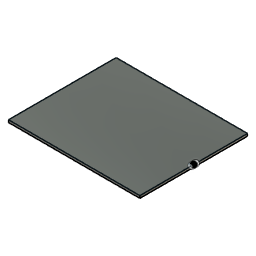
hydraulique (Autodesk Fusion 360 design; units mm, degrees)
Autodesk Fusion 360 part; units mm, degrees
box "BoxPrimitive1" add length 136 width 166 height 3 placed x (0, -1, 0) y (1, 0, 0) z (0, 0, 1) at (-30, 40, 0)
move_body "Move1" bodies 1 to x (1, 0, 0) y (0, 1, 0) z (0, 0, 1) at (-59.3373, 23.0424, 23.0424)
move_body "Move2" bodies 1 to x (1, 0, 0) y (0, 1, 0) z (0, 0, 1) at (6.3373, 4.9576, -26.0424)
move_body "Move3" bodies 1 to x (1, 0, 0) y (0, 1, 0) z (0, 0, 1) at (0, 0, 3)
sketch "Sketch6" plane through (0, 0, 3) normal (0, 0, 1) x (-1, 0, 0)
  line L0 (83, 68) -> (-83, 68)
  line L1 (-83, 68) -> (-83, -68)
  line L2 (-83, -68) -> (83, -68)
  line L3 (83, -68) -> (83, 68)
  line L4 (-80.5, -2.5) -> (-83, -2.5)
  line L5 (-83, 2.5) -> (-80.5, 2.5)
  line L6 (-80.5, 2.5) -> (-80.5, -2.5)
  point P0 (-83, 0)
  constraint midpoint L1 P0
  constraint horizontal L4
  constraint horizontal L5
  constraint vertical L6
extrude "Extrude2" cut sketch "Sketch6" against normal blind 3 contours L1 L4 L5 L6
